endfeedconnector (Autodesk Fusion 360 design; units mm, degrees)
Autodesk Fusion 360 part; units mm, degrees
note: some values were not read from the file. Chosen so that the rebuilt part matches the saved one: which face or edge a step refers to; which pieces of a blend or face edit are solid.
sketch "Sketch1" plane through (0, 0, 0) normal (0, 0, 1) x (1, 0, 0)
  circle A0 centre (0, 0) radius 8.5
  circle A1 centre (0, 0) radius 10.5
  circle A2 centre (0, 0) radius 4.5
  circle A3 centre (0, 0) radius 3
  arc A4 (0.9668, 2.84) -> (-1.1676, 2.7635) centre (-0.1074, 2.9981) ccw
  dimension "d1" = 17
  dimension "d2" = 21
  dimension "d3" = 9
  dimension "d4" = 6
  dimension "d12" = 17
  constraint coincident A0.centre A1.centre
  constraint concentric A0 A1
  constraint concentric A1 A2
  constraint concentric A2 A3
  constraint coincident A3 A4.centre
  constraint coincident A3 A4.end
  constraint coincident A3 A4.start
  measures "d1" diameter of A0
  measures "d2" diameter of A1
  measures "d3" diameter of A2
  measures "d4" diameter of A3
  measures "d12" diameter of A0
extrude "Extrude1" add sketch "Sketch1" against normal blind 12 contours A2 | A3 | A3 A4
extrude "Extrude2" add sketch "Sketch1" along normal blind 12 contours A0 | A1 | A2 | A3 A4
extrude "Extrude3" cut sketch "Sketch1" against normal blind 24 contours A3
ref_plane "WorkPlane1" through (0, 0, 15) normal (0, 0, 1) x (1, 0, 0)
sketch "Sketch2" plane through (0, 0, 15) normal (0, 0, 1) x (1, 0, 0)
  circle A0 centre (0, 0) radius 8.5
  dimension "d13" = 17
  constraint coincident A0.centre origin
  measures "d13" diameter of A0
extrude "Extrude4" cut sketch "Sketch2" against normal blind 10
sketch "Sketch3" plane through (0, 0, 0) normal (1, 0, 0) x (0, 1, 0)
  circle A0 centre (0, 10) radius 0.8
  dimension "d16" = 1.6
  measures "d16" diameter of A0
extrude "Extrude5" cut sketch "Sketch3" along normal mid plane 30
chamfer "Chamfer1" distance 6 angle 45 1 edges at (-4.1955, -1.6273, 0)
fillet "Fillet1" radius 3 2 edges at (-10.4988, 0, 0) (-10.5, 0, 0)
extrude "Extrude6" cut sketch "Sketch1" along normal mid plane 28 contours A3 A4
